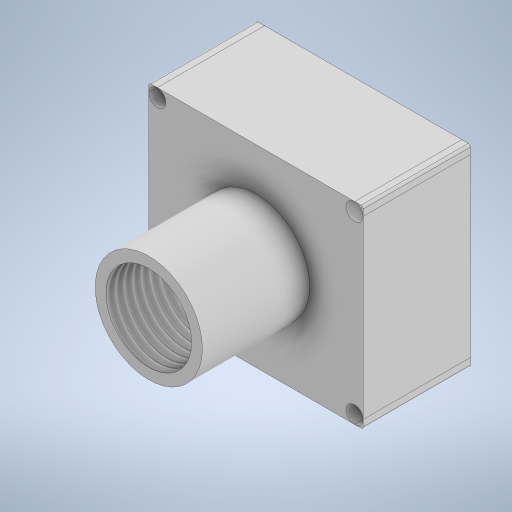
# Autodesk Inventor part: Práctica1
Saved by Autodesk Inventor 2024 (Build 280153000, 153)
## iProperties
Created: 2024-02-19
Part Number: Práctica1
Material: Generic
Document SubType Name: Modeling
Designer: Ian
Density: 1 g/cm^3
Appearance: Default
Author: Ian
Autodesk Inventor part; units mm, degrees
ref_plane "YZ Plane" through (0, 0, 0) normal (1, 0, 0) x (0, 1, 0)
ref_plane "XZ Plane" through (0, 0, 0) normal (0, 1, 0) x (-1, 0, 0)
ref_plane "XY Plane" through (0, 0, 0) normal (0, 0, 1) x (1, 0, 0)
sketch "Sketch1" plane through (0, 0, 0) normal (0, 0, 1) x (1, 0, 0)
  line L0 (50, -45) -> (-50, -45)
  line L1 (-50, -45) -> (-50, 45)
  line L2 (-50, 45) -> (50, 45)
  line L3 (50, 45) -> (50, -45)
  line L4 (50, -45) -> (-50, 45) construction
  line L5 (-50, -45) -> (50, 45) construction
  point P0 (0, 0)
  dimension "d0" = 100
  dimension "d1" = 90
  constraints: 12 end point, 2 midpoint, 2 parallel, 1 horizontal, 1 perpendicular
  measures "d0" distance of L1.end L2.end
  measures "d1" distance of L0.end L1.end
extrude "Extrusion1" add sketch "Sketch1" along normal blind 50
sketch "Sketch2" plane through (0, 0, 50) normal (0, 0, 1) x (1, 0, 0)
  line L0 (50, -45) -> (50, 45) projected
  line L1 (50, 45) -> (-50, 45) projected
  circle A0 centre (46, 41) radius 4
  circle A1 centre (-46, 41) radius 4
  line L2 (-50, 45) -> (-50, -45) projected
  circle A2 centre (-46, -41) radius 4
  line L3 (-50, -45) -> (50, -45) projected
  circle A3 centre (46, -41) radius 4
  point P0 (0, 0)
  constraints: 8 tangent, 4 centre point
extrude "Extrusion2" cut sketch "Sketch2" against normal through all contours A3 | A0 | A2 | A1
sketch "Sketch3" plane through (0, 0, 50) normal (0, 0, 1) x (1, 0, 0)
  circle A0 centre (0, 0) radius 25
  circle A1 centre (0, 0) radius 20
  constraints: 2 centre point, 2 coincident
extrude "Extrusion3" add sketch "Sketch3" along normal blind 50
thread "Thread1" size "M50x4" class "6H" standard "ANSI Metric M Profile" length 30
fillet "Fillet1" radius 1 1 edges at (50, 45, 25)
fillet "Fillet2" radius 1 3 edges at (50, -45, 25) (-50, -45, 25) (-50, 45, 25)
body "Solid1"
